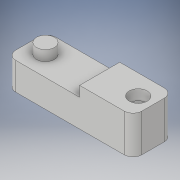
# Autodesk Inventor part: Shoulder2 Link
Saved by Autodesk Inventor 2017 (Build 210142000, 142)
## iProperties
Created: 2017-05-25
Part Number: Shoulder2 Link
Material: Generic
Document SubType Name: Modeling
Designer: garre
Density: 1 g/cm^3
Appearance: Default
Author: garre
Autodesk Inventor part; units mm, degrees
ref_plane "YZ Plane" through (0, 0, 0) normal (1, 0, 0) x (0, 1, 0)
ref_plane "XZ Plane" through (0, 0, 0) normal (0, 1, 0) x (-1, 0, 0)
ref_plane "XY Plane" through (0, 0, 0) normal (0, 0, 1) x (1, 0, 0)
sketch "Sketch1" plane through (0, 0, 0) normal (0, 1, 0) x (-1, 0, 0)
  circle A0 centre (0, 0) radius 30.734
  line L0 (-20.32, 68.58) -> (350.52, 68.58)
  line L1 (381, 38.1) -> (381, -38.1)
  line L2 (350.52, -68.58) -> (-20.32, -68.58)
  line L3 (-50.8, -38.1) -> (-50.8, 38.1)
  arc A1 (-20.32, 68.58) -> (-50.8, 38.1) centre (-20.32, 38.1) ccw
  arc A2 (-50.8, -38.1) -> (-20.32, -68.58) centre (-20.32, -38.1) ccw
  arc A3 (381, 38.1) -> (350.52, 68.58) centre (350.52, 38.1) ccw
  arc A4 (350.52, -68.58) -> (381, -38.1) centre (350.52, -38.1) ccw
  point P0 (-50.8, 68.58)
  point P1 (381, -68.58)
  point P2 (-50.8, -68.58)
  dimension "d0" = 61.468
  dimension "d1" = 137.16
  dimension "d2" = 431.8
  dimension "d3" = 50.8
  dimension "d4" = 68.58
  dimension "d5" = 30.48
  constraints: 8 end point, 8 point on circle, 8 tangent, 6 point on line, 5 centre point, 3 equal radius, 2 parallel, 1 coincident, 1 horizontal, 1 perpendicular
  measures "d0" diameter of A0
  measures "d1" distance of point (-50.8, -68.58) point (-50.8, 68.58)
  measures "d2" distance of point (381, -68.58) point (-50.8, -68.58)
  measures "d3" distance from line of L3 point (0, 0)
  measures "d4" distance from line of L2 point (0, 0)
  measures "d5" radius of A1
extrude "Extrusion1" add sketch "Sketch1" against normal blind 129.54
sketch "Sketch2" plane through (0, -129.54, 0) normal (0, -1, 0) x (1, 0, 0)
  circle A0 centre (0, 0) radius 38.1
  dimension "d17" = 76.2
  constraints: 1 centre point, 1 coincident
  measures "d17" diameter of A0
extrude "Extrusion2" add sketch "Sketch2" against normal blind 93.98
sketch "Sketch3" plane through (0, 0, 0) normal (0, 1, 0) x (1, 0, 0)
  line L0 (50.8, 38.1) -> (50.8, -38.1) projected
  line L1 (50.8, 0) -> (-132.08, 0)
  line L2 (20.32, -68.58) -> (-350.52, -68.58) projected
  line L3 (-132.08, -68.58) -> (-434.975, -68.58)
  line L4 (-434.975, -68.58) -> (-434.975, 68.58)
  line L5 (-434.975, 68.58) -> (-132.08, 68.58)
  line L6 (-132.08, 68.58) -> (-132.08, -68.58)
  point P0 (0, 0)
  dimension "d10" = 182.88
  constraints: 10 end point, 2 horizontal, 2 parallel, 1 midpoint, 1 perpendicular, 1 point on line
  measures "d10" distance of L1.start L1.end
extrude "Extrusion3" cut sketch "Sketch3" against normal blind 35.2425
sketch "Sketch4" plane through (0, -35.2425, 0) normal (0, 1, 0) x (1, 0, 0)
  line L0 (-381, -38.1) -> (-381, 38.1) projected
  line L1 (-381, 0) -> (-328.6125, 0)
  line L2 (-381, 0) -> (-317.5, 0)
  circle A0 centre (-317.5, 0) radius 30.48
  point P0 (0, 0)
  dimension "d14" = 60.96
  dimension "d18" = 317.5
  constraints: 4 end point, 1 centre point, 1 coincident, 1 horizontal, 1 midpoint, 1 point on line
  measures "d14" diameter of A0
  measures "d18" distance of point (0, 0) L2.end
extrude "Extrusion4" add sketch "Sketch4" along normal blind 35.56
equation "\"d4\" = 0.5 * d1"
body "Solid1"
